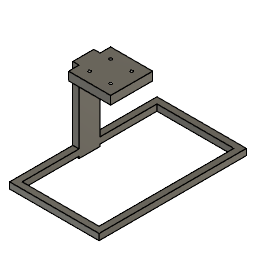
Y Axis Mount (Autodesk Fusion 360 design; units mm, degrees)
Autodesk Fusion 360 part; units mm, degrees
note: some values were not read from the file. Set by a fixed rule: the direction of a hole.
sketch "Sketch1" plane through (0, 0, 0) normal (0, 0, 1) x (1, 0, 0)
  line L0 (20, -20) -> (-20, -20)
  line L1 (-20, -20) -> (-20, 20)
  line L2 (-20, 20) -> (20, 20)
  line L3 (20, 20) -> (20, -20)
  line L4 (20, -20) -> (-20, 20) construction
  line L5 (-20, -20) -> (20, 20) construction
  point P0 (-10, 10)
  point P1 (10, -10)
  point P2 (-10, -10)
  point P3 (10, 10)
  dimension "d1" = 40
  dimension "d2" = 40
  dimension "d3" = 10
  dimension "d4" = 10
  constraint horizontal L0
  constraint perpendicular L0 L1
  constraint parallel L0 L2
  constraint parallel L1 L3
  constraint coincident L4 origin
  constraint coincident L5 origin
  constraint coincident L4 P1
  constraint coincident L5 P2
  constraint coincident L5 P3
  constraint horizontal P0 P3
  constraint vertical P0 P2
  constraint vertical P1 P3
  measures "d1" distance of L1.end L2.end
  measures "d2" distance of L0.end L1.end
  measures "d3" distance of L1 P0
  measures "d4" distance of L2 P0
extrude "Extrude1" add sketch "Sketch1" along normal blind 8
hole "Hole1" at (-10, 10, 0) at (10, 10, 0) at (10, -10, 0) at (-10, -10, 0) direction (0, 0, 1) diameter 2.529 depth 40 tip angle 118
thread "Thread1" "ISO Metric profile 3.0 M3x0.5 M3x0.5 6H" major diameter 3.086 minor diameter 2.529 pitch 0.5 angle 60 resizes the face on face at (10.1259, -8.7418, 5.3333) on face at (10.1259, 11.2582, 5.3333) on face at (-9.8741, 11.2582, 5.3333) on face at (-9.8741, -8.7418, 5.3333)
sketch "Sketch2" plane through (0, 0, 8) normal (0, 0, 1) x (-1, 0, 0)
  circle A0 centre (-10, 10) radius 1.2645
  circle A1 centre (10, -10) radius 1.2645
  circle A2 centre (-10, -10) radius 1.2645
  circle A3 centre (10, 10) radius 1.2645
  line L0 (-20, -20) -> (20, -20)
  line L1 (20, -20) -> (20, 20)
  line L2 (20, 20) -> (-20, 20)
  line L3 (-20, 20) -> (-20, -20)
  line L4 (20, -10) -> (26, -10)
  line L5 (26, -10) -> (26, 10)
  line L6 (26, 10) -> (20, 10)
  line L7 (20, 10) -> (20, -10)
  dimension "d13" = 6
  dimension "d14" = 20
  dimension "d15" = 10
  constraint horizontal L4
  constraint vertical L5
  constraint horizontal L6
  constraint vertical L7
  constraint coincident L1 L4.start
  measures "d13" distance of L4.start L4.end
  measures "d14" distance of L4.start L6.end
  measures "d15" distance of L0.end L4.start
extrude "Extrude2" add sketch "Sketch2" against normal blind 75 contours L1 L4 L5 L6 L7
sketch "Sketch3" plane through (0, 0, -67) normal (0, 0, -1) x (1, 0, 0)
  line L0 (-20, -10) -> (-20, 10)
  line L1 (-20, 10) -> (-26, 10)
  line L2 (-26, 10) -> (-26, -10)
  line L3 (-26, -10) -> (-20, -10)
  line L4 (-20, -64) -> (53, -64)
  line L5 (53, -64) -> (53, 64)
  line L6 (53, 64) -> (-20, 64)
  line L7 (-20, 64) -> (-20, -64)
  line L8 (-20, -20) -> (-20, -10)
  line L9 (59, 70) -> (-26, 70)
  line L10 (-26, 70) -> (-26, -70)
  line L11 (-26, -70) -> (59, -70)
  line L12 (59, -70) -> (59, 70)
  dimension "d24" = 73
  dimension "d25" = 128
  dimension "d26" = 54
  dimension "d28" = 6
  dimension "d29" = 6
  constraint horizontal L4
  constraint vertical L5
  constraint horizontal L6
  constraint vertical L7
  measures "d24" distance of L4.start L4.end
  measures "d25" distance of L4.start L6.end
  measures "d26" vertical distance of L2.end L4.start
  measures "d28" distance of L2 L7
extrude "Extrude3" add sketch "Sketch3" along normal mid plane 4 contours L0 L1 L2 L3 L7 L10
extrude "Extrude4" add sketch "Sketch3" against normal blind 6 contours L1 L3 L4 L5 L6 L7 L8 L9 L10 L11 L12
equation "d26 = ( ( 128 - 20 ) / 2 ) * 1 mm"
